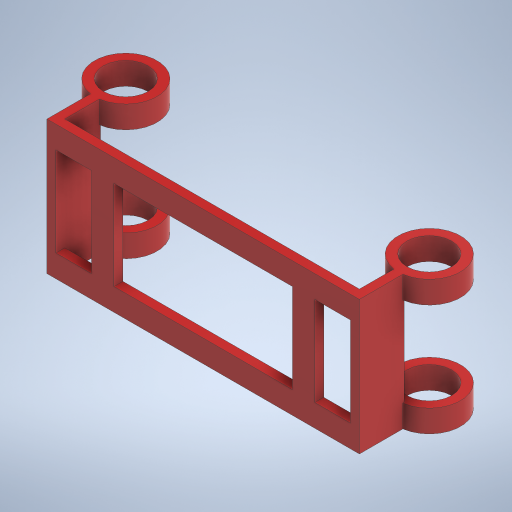
# Autodesk Inventor part: Slider 10mm
Saved by Autodesk Inventor 2024 (Build 280153000, 153)
## iProperties
Created: 2023-09-10
Part Number: Slider 10mm
Material: Generic
Document SubType Name: Modeling
Designer: AlfaNooraFithria
Density: 1 g/cm^3
Appearance: Default
Author: AlfaNooraFithria
Autodesk Inventor part; units mm, degrees
ref_plane "YZ Plane" through (0, 0, 0) normal (1, 0, 0) x (0, 1, 0)
sketch "Sketch1" plane through (0, 0, 0) normal (0, 0, 1) x (1, 0, 0)
  line L0 (0, 0) -> (70, 0)
  line L1 (70, 0) -> (70, 30)
  line L2 (70, 30) -> (0, 30)
  line L3 (0, 30) -> (0, 0)
  line L4 (55, 15) -> (55, 25)
  line L5 (55, 25) -> (35, 25)
  line L6 (68, 15) -> (68, 25)
  line L7 (68, 25) -> (60, 25)
  line L8 (60, 25) -> (60, 15)
  line L9 (15, 15) -> (15, 25)
  line L10 (15, 25) -> (35, 25)
  line L11 (2, 15) -> (2, 25)
  line L12 (2, 25) -> (10, 25)
  line L13 (10, 25) -> (10, 15)
  line L14 (55, 15) -> (55, 5)
  line L15 (55, 5) -> (35, 5)
  line L16 (68, 15) -> (68, 5)
  line L17 (68, 5) -> (60, 5)
  line L18 (60, 5) -> (60, 15)
  line L19 (15, 5) -> (35, 5)
  line L20 (15, 15) -> (15, 5)
  line L21 (10, 5) -> (10, 15)
  line L22 (2, 5) -> (10, 5)
  line L23 (2, 15) -> (2, 5)
  dimension "d0" = 70
  dimension "d1" = 30
  dimension "d2" = 20
  dimension "d3" = 10
  dimension "d5" = 8
  constraints: 48 end point, 3 parallel, 1 horizontal, 1 perpendicular
  measures "d0" distance of L2.end L1.end
  measures "d1" distance of L1.end L0.end
  measures "d2" distance of L5.end L4.end
  measures "d3" distance of L4.end L4.start
  measures "d5" distance of L7.end L6.end
extrude "Extrusion1" add sketch "Sketch1" against normal blind 10
sketch "Sketch2" plane through (0, 0, -10) normal (0, 0, -1) x (-1, 0, 0)
  line L0 (-70, 30) -> (-70, 0) projected
  line L1 (-70, 30) -> (0, 30)
  line L2 (0, 30) -> (0, 0)
  line L3 (0, 0) -> (-70, 0)
  line L4 (-70, 0) -> (-70, 30)
  line L5 (-68, 28) -> (-68, 2)
  line L6 (-2, 2) -> (-2, 28)
  line L7 (-68, 28) -> (-68, 30)
  line L8 (-70, 30) -> (0, 30) projected
  line L9 (-68, 2) -> (-68, 0)
  line L10 (-2, 2) -> (-2, 0)
  line L11 (-2, 28) -> (-2, 30)
  line L12 (-68, 30) -> (-2, 30)
  line L13 (-2, 30) -> (-2, 0)
  line L14 (-2, 0) -> (-68, 0)
  line L15 (-68, 0) -> (-68, 30)
  constraints: 28 end point, 6 point on line, 5 parallel, 4 perpendicular, 2 horizontal
extrude "Extrusion2" cut sketch "Sketch2" against normal blind 8 contours L1 L11 L6 L10 L3 L9 L5 L7
sketch "Sketch3" plane through (0, 30, 0) normal (0, 1, 0) x (1, 0, 0)
  line L0 (0, 10) -> (2, 10) projected
  circle A0 centre (1, 16.6661) radius 5
  circle A1 centre (1, 16.6661) radius 7
  point P0 (0, 0)
  dimension "d11" = 10
  dimension "d12" = 2
  constraints: 2 centre point
  measures "d11" diameter of A0
  measures "d12" radial gap between concentric circles of A0 A1
extrude "Extrusion3" add sketch "Sketch3" against normal blind 5
ref_plane "Work Plane1" through (35, 0, 0) normal (-1, 0, 0) x (0, 0, 1)
ref_plane "Work Plane2" through (0, 15, 0) normal (0, 1, 0) x (1, 0, 0)
mirror "Mirror1" about plane through (0, 15, 0) normal (0, 1, 0) of "Extrusion3"
mirror "Mirror2" about plane through (35, 0, 0) normal (-1, 0, 0) of "Extrusion3", "Mirror1"
body "Solid1"
